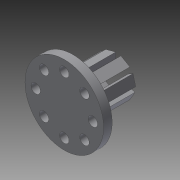
# Autodesk Inventor part: simple_holder
Saved by Autodesk Inventor 2013 (Build 170138000, 138)
## iProperties
Created: 2013-03-18
Part Number: simple_holder
Material: Generic
Document SubType Name: Modeling
Designer: Mahisorn
Density: 1 g/cm^3
Author: Mahisorn
Autodesk Inventor part; units mm, degrees
ref_plane "YZ Plane" through (0, 0, 0) normal (1, 0, 0) x (0, 1, 0)
ref_plane "XZ Plane" through (0, 0, 0) normal (0, 1, 0) x (-1, 0, 0)
ref_plane "XY Plane" through (0, 0, 0) normal (0, 0, 1) x (1, 0, 0)
sketch "Sketch7" plane through (0, 0, 0) normal (0, 1, 0) x (-1, 0, 0)
  circle A0 centre (0, 0) radius 27.5
  dimension "d35" = 55
  constraints: 1 centre point, 1 coincident
  measures "d35" diameter of A0
extrude "Extrusion5" add sketch "Sketch7" along normal blind 6
sketch "Sketch8" plane through (0, 6, 0) normal (0, 1, 0) x (1, 0, 0)
  circle A0 centre (0, 0) radius 27.5 projected
  point P0 (20, 0)
  point P1 (14.1421, 14.1421)
  point P2 (0, 20)
  point P3 (-14.1421, 14.1421)
  point P4 (-20, 0)
  point P5 (-14.1421, -14.1421)
  point P6 (0, -20)
  point P7 (14.1421, -14.1421)
  dimension "d38" = 20
  dimension "d41" = 360
  constraints: 9 other
  measures "d38" distance of A0.centre point (20, 0)
hole "Hole2" at (20, 6, 0) at (14.1421, 6, -14.1421) at (0, 6, -20) at (-14.1421, 6, -14.1421) at (-20, 6, 0) at (-14.1421, 6, 14.1421) at (0, 6, 20) at (14.1421, 6, 14.1421) direction (0, -1, 0) diameter 6.6 end through all clearance for "Flat Head Machine Screw" size "M6" standard "Ansi Metric M Profile"
sketch "Sketch9" plane through (0, 6, 0) normal (0, 1, 0) x (1, 0, 0)
  circle A0 centre (0, 0) radius 27.5 projected
  line L0 (-14, 0) -> (-10, 0)
  line L1 (-8.6603, 5) -> (-10, 0)
  line L2 (-12.1244, 7) -> (-14, 0)
  line L3 (-12.1244, 7) -> (-8.6603, 5)
  dimension "d59" = 4
  dimension "d60" = 10
  constraints: 8 end point, 1 horizontal, 1 parallel
  measures "d59" distance of L0.start L0.end
  measures "d60" distance of A0.centre L0.end
extrude "Extrusion6" add sketch "Sketch9" along normal blind 30 contours L2 L3 L1 L0
fillet "Fillet4" radius 0.5 3 edges at (-12, 6, 0) (-10.3923, 6, -6) (-13.0622, 6, -3.5)
fillet "Fillet5" radius 3 3 edges at (-10.067, 6, 0.25) (-9.3301, 6, -2.5) (-8.5933, 6, -5.25)
pattern_circular "Circular Pattern1" count 8 over 360 about axis through (0, 0, 0) along (0, 1, 0) of "Extrusion6", "Fillet4", "Fillet5"
body "Solid2"
